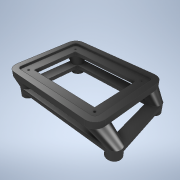
# Autodesk Inventor part: Suporte_ESP32
Saved by Autodesk Inventor 2020 (Build 240168000, 168)
## iProperties
Created: 2022-05-24
Part Number: Suporte_ESP32
Material: Genérico
Document SubType Name: Modeling
Designer: JCarlos
Density: 1 g/cm^3
Appearance: Brilhosa - Preta
Author: JCarlos
Autodesk Inventor part; units mm, degrees
ref_plane "YZ Plane" through (0, 0, 0) normal (1, 0, 0) x (0, 1, 0)
ref_plane "XZ Plane" through (0, 0, 0) normal (0, 1, 0) x (-1, 0, 0)
sketch "Esboço1" plane through (0, 0, 0) normal (0, 1, 0) x (-1, 0, 0)
  line L0 (34.5, -27.5) -> (-34.5, -27.5)
  line L1 (-37.5, -24.5) -> (-37.5, 24.5)
  line L2 (-34.5, 27.5) -> (34.5, 27.5)
  line L3 (37.5, 24.5) -> (37.5, -24.5)
  arc A0 (34.5, -27.5) -> (37.5, -24.5) centre (34.5, -24.5) ccw
  arc A1 (37.5, 24.5) -> (34.5, 27.5) centre (34.5, 24.5) ccw
  arc A2 (-34.5, 27.5) -> (-37.5, 24.5) centre (-34.5, 24.5) ccw
  arc A3 (-37.5, -24.5) -> (-34.5, -27.5) centre (-34.5, -24.5) ccw
  line L4 (-34.5, -32.5) -> (34.5, -32.5)
  arc A4 (34.5, -32.5) -> (42.5, -24.5) centre (34.5, -24.5) ccw
  line L5 (42.5, -24.5) -> (42.5, 24.5)
  arc A5 (42.5, 24.5) -> (34.5, 32.5) centre (34.5, 24.5) ccw
  line L6 (34.5, 32.5) -> (-34.5, 32.5)
  arc A6 (-34.5, 32.5) -> (-42.5, 24.5) centre (-34.5, 24.5) ccw
  line L7 (-42.5, 24.5) -> (-42.5, -24.5)
  arc A7 (-42.5, -24.5) -> (-34.5, -32.5) centre (-34.5, -24.5) ccw
  point P0 (0, 0)
  point P1 (37.5, -27.5)
  point P2 (-37.5, -27.5)
  point P3 (37.5, 27.5)
  point P4 (37.5, 0)
  point P5 (0, -27.5)
  dimension "d0" = 75
  dimension "d1" = 55
  dimension "d2" = 3
  dimension "d4" = 5
  constraints: 16 end point, 16 point on circle, 8 centre point, 8 tangent, 6 point on line, 4 parallel, 3 equal radius, 2 midpoint, 2 perpendicular, 1 horizontal, 1 horizontal alignment, 1 vertical alignment, 23 other
  measures "d0" distance of point (37.5, -27.5) point (-37.5, -27.5)
  measures "d1" distance of point (37.5, 27.5) point (37.5, -27.5)
  measures "d2" radius of A0
  measures "d4" distance between parallel lines of L4 L0
extrude "Extrusão1" add sketch "Esboço1" along normal blind 5
sketch "Esboço2" plane through (0, 0, 0) normal (0, -1, 0) x (1, 0, 0)
  line L0 (-42.5, -24.5) -> (-42.5, 24.5) projected
  arc A0 (-42.5, -24.5) -> (-34.5, -32.5) centre (-34.5, -24.5) ccw projected
  line L1 (34.5, -32.5) -> (-34.5, -32.5) projected
  arc A1 (34.5, -32.5) -> (42.5, -24.5) centre (34.5, -24.5) ccw projected
  line L2 (42.5, 24.5) -> (42.5, -24.5) projected
  arc A2 (42.5, 24.5) -> (34.5, 32.5) centre (34.5, 24.5) ccw projected
  line L3 (-34.5, 32.5) -> (34.5, 32.5) projected
  arc A3 (-34.5, 32.5) -> (-42.5, 24.5) centre (-34.5, 24.5) ccw projected
  arc A4 (37.5, 24.5) -> (34.5, 27.5) centre (34.5, 24.5) ccw projected
  line L4 (37.5, -24.5) -> (37.5, 24.5) projected
  arc A5 (34.5, -27.5) -> (37.5, -24.5) centre (34.5, -24.5) ccw projected
  line L5 (-34.5, -27.5) -> (34.5, -27.5) projected
  arc A6 (-37.5, -24.5) -> (-34.5, -27.5) centre (-34.5, -24.5) ccw projected
  line L6 (-37.5, 24.5) -> (-37.5, -24.5) projected
  arc A7 (-34.5, 27.5) -> (-37.5, 24.5) centre (-34.5, 24.5) ccw projected
  line L7 (34.5, 27.5) -> (-34.5, 27.5) projected
  line L8 (29.5, 19.5) -> (-29.5, 19.5)
  line L9 (-29.5, 19.5) -> (-29.5, -19.5)
  line L10 (-29.5, -19.5) -> (29.5, -19.5)
  line L11 (29.5, -19.5) -> (29.5, 19.5)
  point P0 (0, 0)
  dimension "d7" = 8
  constraints: 8 end point, 3 other
  measures "d7" distance between parallel lines of L4 L11
extrude "Extrusão2" add sketch "Esboço2" against normal blind 3 contours L4 A5 L5 A6 L6 A7 L7 A4
ref_plane "Plano de trabalho1" through (0, -12, 0) normal (0, 1, 0) x (1, 0, 0)
sketch "Esboço3" plane through (0, -12, 0) normal (0, 1, 0) x (1, 0, 0)
  circle A0 centre (49.5, -24.15) radius 1 projected
  circle A1 centre (49.5, -24.15) radius 3 projected
  circle A2 centre (43, 24.1) radius 1 projected
  circle A3 centre (43, 24.1) radius 3 projected
  circle A4 centre (-33, -24.15) radius 1 projected
  circle A5 centre (-33, -24.15) radius 3 projected
  circle A6 centre (-32, 24.1) radius 1 projected
  circle A7 centre (-32, 24.1) radius 3 projected
  circle A8 centre (43, 24.1) radius 3.5
  circle A9 centre (43, 24.1) radius 5.5
  circle A10 centre (-32, 24.1) radius 3.5
  circle A11 centre (-32, 24.1) radius 5.5
  circle A12 centre (-33, -24.15) radius 3.5
  circle A13 centre (-33, -24.15) radius 5.5
  circle A14 centre (49.5, -24.15) radius 3.5
  circle A15 centre (49.5, -24.15) radius 5.5
  point P0 (0, 0)
  dimension "d11" = 0.5
  dimension "d12" = 2
  dimension "d13" = 2
  dimension "d14" = 2
  dimension "d15" = 2
  dimension "d18" = 0.5
  dimension "d19" = 0.5
  dimension "d20" = 0.5
  constraints: 8 centre point, 3 equal radius
  measures "d11" radial gap between concentric circles of A3 A8
  measures "d12" radial gap between concentric circles of A8 A9
  measures "d13" radial gap between concentric circles of A10 A11
  measures "d14" radial gap between concentric circles of A12 A13
  measures "d15" radial gap between concentric circles of A14 A15
  measures "d18" radial gap between concentric circles of A14 A1
  measures "d19" radial gap between concentric circles of A12 A5
  measures "d20" radial gap between concentric circles of A10 A7
extrude "Extrusão3" add sketch "Esboço3" against normal blind 5 contours A9 | A11 | A13 | A15
sketch "Esboço4" plane through (0, -12, 0) normal (0, 1, 0) x (1, 0, 0)
  line L0 (-37.4988, 24.214) -> (-38.4988, -24.036)
  line L1 (-33, -29.65) -> (49.5, -29.65)
  line L2 (48.4508, 24.8343) -> (54.9508, -23.4157)
  line L3 (43, 29.6) -> (-32, 29.6)
  arc A0 (-38.4988, -24.036) -> (-33, -29.65) centre (-33, -24.15) ccw
  circle A1 centre (-32, 24.1) radius 5.5 projected
  arc A2 (-32, 29.6) -> (-37.4988, 24.214) centre (-32, 24.1) ccw
  arc A3 (48.4508, 24.8343) -> (43, 29.6) centre (43, 24.1) ccw
  arc A4 (49.5, -29.65) -> (54.9508, -23.4157) centre (49.5, -24.15) ccw
  circle A5 centre (-33, -24.15) radius 5.5 projected
  circle A6 centre (49.5, -24.15) radius 5.5 projected
  circle A7 centre (43, 24.1) radius 5.5 projected
  line L4 (-28.1514, 20.1708) -> (39.5647, 20.1708)
  line L5 (39.5647, 20.1708) -> (45.006, -20.2208)
  line L6 (45.006, -20.2208) -> (-28.9885, -20.2208)
  line L7 (-28.9885, -20.2208) -> (-28.1514, 20.1708)
  point P0 (0, 0)
  constraints: 16 end point, 10 point on circle, 7 tangent, 6 coincident, 4 centre point, 3 concentric, 1 horizontal, 7 other
extrude "Extrusão4" add sketch "Esboço4" along normal blind 3 contours A1 L7 L6 L5 A7 L2 A6 L1 A5 L0 | A1 | A5 A0 | L3 A7 L4 A1 | A3 A7 L5 L4 | A6 A4
sketch "Esboço5" plane through (0, -9, 0) normal (0, 1, 0) x (1, 0, 0)
  circle A0 centre (49.5, -24.15) radius 5.5
  arc A1 (49.5, -29.65) -> (54.9508, -23.4157) centre (49.5, -24.15) ccw projected
  point P0 (0, 0)
  constraints: 2 concentric, 1 centre point, 1 coincident
sketch "Esboço6" plane through (0, 0, 0) normal (0, -1, 0) x (1, 0, 0)
  circle A0 centre (34.5, 24.5) radius 8
  arc A1 (42.5, 24.5) -> (34.5, 32.5) centre (34.5, 24.5) ccw projected
  point P0 (0, 0)
  constraints: 2 concentric, 1 centre point
loft "Transição1" add profiles "Esboço5", "Esboço6"
sketch "Esboço7" plane through (0, 0, 0) normal (0, -1, 0) x (1, 0, 0)
  arc A0 (-34.5, 32.5) -> (-42.5, 24.5) centre (-34.5, 24.5) ccw projected
  circle A1 centre (-34.5, -24.5) radius 8
  arc A2 (-42.5, -24.5) -> (-34.5, -32.5) centre (-34.5, -24.5) ccw projected
  arc A3 (34.5, -32.5) -> (42.5, -24.5) centre (34.5, -24.5) ccw projected
  point P0 (0, 0)
  constraints: 2 concentric, 1 centre point
sketch "Esboço8" plane through (0, -9, 0) normal (0, 1, 0) x (1, 0, 0)
  arc A0 (48.4508, 24.8343) -> (43, 29.6) centre (43, 24.1) ccw projected
  circle A1 centre (-32, 24.1) radius 5.5
  arc A2 (-32, 29.6) -> (-37.4988, 24.214) centre (-32, 24.1) ccw projected
  arc A3 (-38.4988, -24.036) -> (-33, -29.65) centre (-33, -24.15) ccw projected
  point P0 (0, 0)
  constraints: 2 concentric, 1 centre point
loft "Transição2" add profiles "Esboço8", "Esboço7"
sketch "Esboço9" plane through (0, -9, 0) normal (0, 1, 0) x (1, 0, 0)
  circle A0 centre (43, 24.1) radius 5.5
  arc A1 (48.4508, 24.8343) -> (43, 29.6) centre (43, 24.1) ccw projected
  point P0 (0, 0)
  constraints: 2 concentric, 1 centre point
sketch "Esboço10" plane through (0, 0, 0) normal (0, -1, 0) x (1, 0, 0)
  circle A0 centre (34.5, -24.5) radius 8
  arc A1 (34.5, -32.5) -> (42.5, -24.5) centre (34.5, -24.5) ccw projected
  point P0 (0, 0)
  constraints: 2 concentric, 1 centre point
loft "Transição3" add profiles "Esboço9", "Esboço10"
sketch "Esboço11" plane through (0, -9, 0) normal (0, 1, 0) x (1, 0, 0)
  circle A0 centre (-33, -24.15) radius 5.5
  arc A1 (-38.4988, -24.036) -> (-33, -29.65) centre (-33, -24.15) ccw projected
  point P0 (0, 0)
  constraints: 2 concentric, 1 centre point
sketch "Esboço12" plane through (0, 0, 0) normal (0, -1, 0) x (1, 0, 0)
  circle A0 centre (-34.5, 24.5) radius 8
  arc A1 (-34.5, 32.5) -> (-42.5, 24.5) centre (-34.5, 24.5) ccw projected
  point P0 (0, 0)
  constraints: 2 concentric, 1 centre point
loft "Transição4" add profiles "Esboço12", "Esboço11"
sketch "Esboço14" plane through (0, 3, 0) normal (0, 1, 0) x (1, 0, 0)
  circle A0 centre (32.25, 22.25) radius 0.9
  circle A1 centre (32.25, -22.25) radius 0.9
  circle A2 centre (-32.25, 22.25) radius 0.9
  circle A3 centre (-32.25, -22.25) radius 0.9
  point P0 (0, 0)
  dimension "d39" = 44.5
  dimension "d40" = 1.8
  dimension "d41" = 1.8
  dimension "d42" = 22.25
  dimension "d43" = 64.5
  dimension "d44" = 32.25
  constraints: 4 centre point, 2 equal radius, 2 horizontal alignment, 2 vertical alignment
  measures "d39" distance of A1.centre A0.centre
  measures "d40" diameter of A0
  measures "d41" diameter of A1
  measures "d42" vertical distance of A0.centre point (0, 0)
  measures "d43" distance of A0.centre A2.centre
  measures "d44" horizontal distance of point (0, 0) A0.centre
extrude "Extrusão5" cut sketch "Esboço14" against normal blind 5
equation "\"d19\" = d18"
equation "\"d20\" = d19"
equation "\"d41\" = d40"
equation "\"d42\" = 0.5 * d39"
equation "\"d44\" = 0.5 * d43"
